Autodesk Inventor part; units mm, degrees
(part 3 of 3)
  line L948 (-32.5873, 84.3579) -> (-32.5873, 84.1252) construction
  line L949 (-32.5873, 84.1252) -> (-32.5873, 83.9559) construction
  line L950 (-32.5873, 83.9559) -> (-32.6932, 83.8148) construction
  line L951 (-32.6932, 83.8148) -> (-32.8837, 83.7371) construction
  line L952 (-32.8837, 83.7371) -> (-33.7726, 83.3774)
  line L953 (-33.7726, 83.3774) -> (-33.7726, 81.1693)
  line L954 (-34.478, 83.1024) -> (-36.5448, 82.291)
  line L955 (-36.5448, 82.291) -> (-36.5448, 82.2699)
  line L956 (-36.5448, 82.2699) -> (-34.478, 81.4375)
  line L957 (-34.478, 81.4375) -> (-34.478, 83.1024)
  spline S134 degree 3 poles (-36.9188, 84.401) (-37.1445, 84.401) (-37.2785, 84.5491) (-37.2785, 84.782) knots 0 0 0 0 1 1 1 1
  line L958 (-36.9188, 84.401) -> (-37.1445, 84.401) construction
  line L959 (-37.1445, 84.401) -> (-37.2785, 84.5491) construction
  line L960 (-37.2785, 84.5491) -> (-37.2785, 84.782) construction
  line L961 (-37.2785, 84.782) -> (-37.2785, 88.3868)
  spline S135 degree 3 poles (-37.2785, 88.3868) (-37.2785, 88.6195) (-37.1445, 88.7606) (-36.9188, 88.7606) (-36.7, 88.7606) (-36.566, 88.6195) (-36.566, 88.3868) knots 2 2 2 2 3 3 3 4 4 4 4
  line L962 (-37.2785, 88.3868) -> (-37.2785, 88.6195) construction
  line L963 (-37.2785, 88.6195) -> (-37.1445, 88.7606) construction
  line L964 (-37.1445, 88.7606) -> (-36.9188, 88.7606) construction
  line L965 (-36.9188, 88.7606) -> (-36.7, 88.7606) construction
  line L966 (-36.7, 88.7606) -> (-36.566, 88.6195) construction
  line L967 (-36.566, 88.6195) -> (-36.566, 88.3868) construction
  line L968 (-36.566, 88.3868) -> (-36.566, 86.9759)
  line L969 (-36.566, 86.9759) -> (-32.933, 86.9759)
  spline S136 degree 3 poles (-32.933, 86.9759) (-32.7285, 86.9759) (-32.5873, 86.8136) (-32.5873, 86.5879) (-32.5873, 86.3621) (-32.7285, 86.1998) (-32.933, 86.1998) knots 6 6 6 6 7 7 7 8 8 8 8
  line L970 (-32.933, 86.9759) -> (-32.7285, 86.9759) construction
  line L971 (-32.7285, 86.9759) -> (-32.5873, 86.8136) construction
  line L972 (-32.5873, 86.8136) -> (-32.5873, 86.5879) construction
  line L973 (-32.5873, 86.5879) -> (-32.5873, 86.3621) construction
  line L974 (-32.5873, 86.3621) -> (-32.7285, 86.1998) construction
  line L975 (-32.7285, 86.1998) -> (-32.933, 86.1998) construction
  line L976 (-32.933, 86.1998) -> (-36.566, 86.1998)
  line L977 (-36.566, 86.1998) -> (-36.566, 84.775)
  spline S137 degree 3 poles (-36.566, 84.775) (-36.566, 84.5491) (-36.7, 84.401) (-36.9188, 84.401) knots 10 10 10 10 11 11 11 11
  line L978 (-36.566, 84.775) -> (-36.566, 84.5491) construction
  line L979 (-36.566, 84.5491) -> (-36.7, 84.401) construction
  line L980 (-36.7, 84.401) -> (-36.9188, 84.401) construction
  spline S138 degree 3 poles (-34.9648, 88.9871) (-36.3545, 88.9871) (-37.3562, 90.0594) (-37.3562, 91.4562) (-37.3562, 92.853) (-36.3545, 93.9324) (-34.9648, 93.9324) (-33.5679, 93.9324) (-32.5592, 92.853) (-32.5592, 91.4562) (-32.5592, 90.0594) (-33.5679, 88.9871) (-34.9648, 88.9871) knots 0 0 0 0 1 1 1 2 2 2 3 3 3 4 4 4 4
  line L981 (-34.9648, 88.9871) -> (-36.3545, 88.9871) construction
  line L982 (-36.3545, 88.9871) -> (-37.3562, 90.0594) construction
  line L983 (-37.3562, 90.0594) -> (-37.3562, 91.4562) construction
  line L984 (-37.3562, 91.4562) -> (-37.3562, 92.853) construction
  line L985 (-37.3562, 92.853) -> (-36.3545, 93.9324) construction
  line L986 (-36.3545, 93.9324) -> (-34.9648, 93.9324) construction
  line L987 (-34.9648, 93.9324) -> (-33.5679, 93.9324) construction
  line L988 (-33.5679, 93.9324) -> (-32.5592, 92.853) construction
  line L989 (-32.5592, 92.853) -> (-32.5592, 91.4562) construction
  line L990 (-32.5592, 91.4562) -> (-32.5592, 90.0594) construction
  line L991 (-32.5592, 90.0594) -> (-33.5679, 88.9871) construction
  line L992 (-33.5679, 88.9871) -> (-34.9648, 88.9871) construction
  spline S139 degree 3 poles (-33.3211, 91.4562) (-33.3211, 92.3238) (-33.9419, 93.0857) (-34.9577, 93.0857) (-35.9735, 93.0857) (-36.5943, 92.3238) (-36.5943, 91.4562) (-36.5943, 90.5956) (-35.9735, 89.8337) (-34.9577, 89.8337) (-33.9419, 89.8337) (-33.3211, 90.5956) (-33.3211, 91.4562) knots 0 0 0 0 1 1 1 2 2 2 3 3 3 4 4 4 4
  line L993 (-33.3211, 91.4562) -> (-33.3211, 92.3238) construction
  line L994 (-33.3211, 92.3238) -> (-33.9419, 93.0857) construction
  line L995 (-33.9419, 93.0857) -> (-34.9577, 93.0857) construction
  line L996 (-34.9577, 93.0857) -> (-35.9735, 93.0857) construction
  line L997 (-35.9735, 93.0857) -> (-36.5943, 92.3238) construction
  line L998 (-36.5943, 92.3238) -> (-36.5943, 91.4562) construction
  line L999 (-36.5943, 91.4562) -> (-36.5943, 90.5956) construction
  line L1000 (-36.5943, 90.5956) -> (-35.9735, 89.8337) construction
  line L1001 (-35.9735, 89.8337) -> (-34.9577, 89.8337) construction
  line L1002 (-34.9577, 89.8337) -> (-33.9419, 89.8337) construction
  line L1003 (-33.9419, 89.8337) -> (-33.3211, 90.5956) construction
  line L1004 (-33.3211, 90.5956) -> (-33.3211, 91.4562) construction
  line L1005 (-34.3581, 97.4603) -> (-33.2363, 98.582)
  spline S140 degree 3 poles (-33.2363, 98.582) (-33.1518, 98.6737) (-33.067, 98.716) (-32.9613, 98.716) (-32.7778, 98.716) (-32.5873, 98.5467) (-32.5873, 98.3209) (-32.5873, 98.1939) (-32.6438, 98.1094) (-32.7356, 98.0246) knots 1 1 1 1 2 2 2 3 3 3 4 4 4 4
  line L1006 (-33.2363, 98.582) -> (-33.1518, 98.6737) construction
  line L1007 (-33.1518, 98.6737) -> (-33.067, 98.716) construction
  line L1008 (-33.067, 98.716) -> (-32.9613, 98.716) construction
  line L1009 (-32.9613, 98.716) -> (-32.7778, 98.716) construction
  line L1010 (-32.7778, 98.716) -> (-32.5873, 98.5467) construction
  line L1011 (-32.5873, 98.5467) -> (-32.5873, 98.3209) construction
  line L1012 (-32.5873, 98.3209) -> (-32.5873, 98.1939) construction
  line L1013 (-32.5873, 98.1939) -> (-32.6438, 98.1094) construction
  line L1014 (-32.6438, 98.1094) -> (-32.7356, 98.0246) construction
  line L1015 (-32.7356, 98.0246) -> (-34.2523, 96.5715)
  line L1016 (-34.2523, 96.5715) -> (-34.2523, 95.7813)
  line L1017 (-34.2523, 95.7813) -> (-32.933, 95.7813)
  spline S141 degree 3 poles (-32.933, 95.7813) (-32.7215, 95.7813) (-32.5873, 95.6191) (-32.5873, 95.3934) (-32.5873, 95.1676) (-32.7215, 95.0053) (-32.933, 95.0053) knots 7 7 7 7 8 8 8 9 9 9 9
  line L1018 (-32.933, 95.7813) -> (-32.7215, 95.7813) construction
  line L1019 (-32.7215, 95.7813) -> (-32.5873, 95.6191) construction
  line L1020 (-32.5873, 95.6191) -> (-32.5873, 95.3934) construction
  line L1021 (-32.5873, 95.3934) -> (-32.5873, 95.1676) construction
  line L1022 (-32.5873, 95.1676) -> (-32.7215, 95.0053) construction
  line L1023 (-32.7215, 95.0053) -> (-32.933, 95.0053) construction
  line L1024 (-32.933, 95.0053) -> (-36.9471, 95.0053)
  spline S142 degree 3 poles (-36.9471, 95.0053) (-37.1515, 95.0053) (-37.2785, 95.1325) (-37.2785, 95.3581) knots 10 10 10 10 11 11 11 11
  line L1025 (-36.9471, 95.0053) -> (-37.1515, 95.0053) construction
  line L1026 (-37.1515, 95.0053) -> (-37.2785, 95.1325) construction
  line L1027 (-37.2785, 95.1325) -> (-37.2785, 95.3581) construction
  line L1028 (-37.2785, 95.3581) -> (-37.2785, 96.8113)
  spline S143 degree 3 poles (-37.2785, 96.8113) (-37.2785, 98.1094) (-36.5731, 98.6525) (-35.8112, 98.6525) (-35.2398, 98.6525) (-34.5486, 98.2999) (-34.3581, 97.4603) knots 12 12 12 12 13 13 13 14 14 14 14
  line L1029 (-37.2785, 96.8113) -> (-37.2785, 98.1094) construction
  line L1030 (-37.2785, 98.1094) -> (-36.5731, 98.6525) construction
  line L1031 (-36.5731, 98.6525) -> (-35.8112, 98.6525) construction
  line L1032 (-35.8112, 98.6525) -> (-35.2398, 98.6525) construction
  line L1033 (-35.2398, 98.6525) -> (-34.5486, 98.2999) construction
  line L1034 (-34.5486, 98.2999) -> (-34.3581, 97.4603) construction
  spline S144 degree 3 poles (-34.9506, 96.7549) (-34.9506, 97.5309) (-35.3174, 97.806) (-35.7618, 97.806) (-36.1993, 97.806) (-36.566, 97.5309) (-36.566, 96.7549) knots 0 0 0 0 1 1 1 2 2 2 2
  line L1035 (-34.9506, 96.7549) -> (-34.9506, 97.5309) construction
  line L1036 (-34.9506, 97.5309) -> (-35.3174, 97.806) construction
  line L1037 (-35.3174, 97.806) -> (-35.7618, 97.806) construction
  line L1038 (-35.7618, 97.806) -> (-36.1993, 97.806) construction
  line L1039 (-36.1993, 97.806) -> (-36.566, 97.5309) construction
  line L1040 (-36.566, 97.5309) -> (-36.566, 96.7549) construction
  line L1041 (-36.566, 96.7549) -> (-36.566, 95.9224)
  spline S145 degree 3 poles (-36.566, 95.9224) (-36.566, 95.8237) (-36.5237, 95.7813) (-36.4038, 95.7813) knots 3 3 3 3 4 4 4 4
  line L1042 (-36.566, 95.9224) -> (-36.566, 95.8237) construction
  line L1043 (-36.566, 95.8237) -> (-36.5237, 95.7813) construction
  line L1044 (-36.5237, 95.7813) -> (-36.4038, 95.7813) construction
  line L1045 (-36.4038, 95.7813) -> (-34.9506, 95.7813)
  line L1046 (-34.9506, 95.7813) -> (-34.9506, 96.7549)
  spline S146 degree 3 poles (-32.5873, 101.468) (-32.5873, 101.2492) (-32.7215, 101.0801) (-32.933, 101.0801) knots 0 0 0 0 1 1 1 1
  line L1047 (-32.5873, 101.468) -> (-32.5873, 101.2492) construction
  line L1048 (-32.5873, 101.2492) -> (-32.7215, 101.0801) construction
  line L1049 (-32.7215, 101.0801) -> (-32.933, 101.0801) construction
  line L1050 (-32.933, 101.0801) -> (-34.4921, 101.0801)
  line L1051 (-34.4921, 101.0801) -> (-36.693, 99.3446)
  spline S147 degree 3 poles (-36.693, 99.3446) (-36.9612, 99.1329) (-37.3279, 99.3305) (-37.3279, 99.6762) (-37.3279, 99.8314) (-37.2433, 99.9372) (-37.0952, 100.05) knots 3 3 3 3 4 4 4 5 5 5 5
  line L1052 (-36.693, 99.3446) -> (-36.9612, 99.1329) construction
  line L1053 (-36.9612, 99.1329) -> (-37.3279, 99.3305) construction
  line L1054 (-37.3279, 99.3305) -> (-37.3279, 99.6762) construction
  line L1055 (-37.3279, 99.6762) -> (-37.3279, 99.8314) construction
  line L1056 (-37.3279, 99.8314) -> (-37.2433, 99.9372) construction
  line L1057 (-37.2433, 99.9372) -> (-37.0952, 100.05) construction
  line L1058 (-37.0952, 100.05) -> (-35.2752, 101.4751)
  line L1059 (-35.2752, 101.4751) -> (-37.0881, 102.8929)
  spline S148 degree 3 poles (-37.0881, 102.8929) (-37.2363, 103.0129) (-37.3279, 103.0975) (-37.3279, 103.2739) (-37.3279, 103.6196) (-36.9471, 103.81) (-36.6789, 103.5914) knots 7 7 7 7 8 8 8 9 9 9 9
  line L1060 (-37.0881, 102.8929) -> (-37.2363, 103.0129) construction
  line L1061 (-37.2363, 103.0129) -> (-37.3279, 103.0975) construction
  line L1062 (-37.3279, 103.0975) -> (-37.3279, 103.2739) construction
  line L1063 (-37.3279, 103.2739) -> (-37.3279, 103.6196) construction
  line L1064 (-37.3279, 103.6196) -> (-36.9471, 103.81) construction
  line L1065 (-36.9471, 103.81) -> (-36.6789, 103.5914) construction
  line L1066 (-36.6789, 103.5914) -> (-34.4991, 101.8559)
  line L1067 (-34.4991, 101.8559) -> (-32.933, 101.8559)
  spline S149 degree 3 poles (-32.933, 101.8559) (-32.7215, 101.8559) (-32.5873, 101.6797) (-32.5873, 101.468) knots 11 11 11 11 12 12 12 12
  line L1068 (-32.933, 101.8559) -> (-32.7215, 101.8559) construction
  line L1069 (-32.7215, 101.8559) -> (-32.5873, 101.6797) construction
  line L1070 (-32.5873, 101.6797) -> (-32.5873, 101.468) construction
  line L1071 (-53.5384, 32.9027) -> (-44.9652, 32.9027)
  line L1072 (-44.9652, 32.9027) -> (-44.9652, 34.4015)
  line L1073 (-44.9652, 34.4015) -> (-53.5384, 34.4015)
  line L1074 (-53.5384, 34.4015) -> (-53.5384, 32.9027)
  point P0 (0, 0)
  constraints: 452 end point, 2 parallel, 1 horizontal, 1 perpendicular, 434 other
emboss "Emboss1" sketch "Sketch6" operation cut depth 0.5 direction (0, -1, 0)
body "Solid1"
